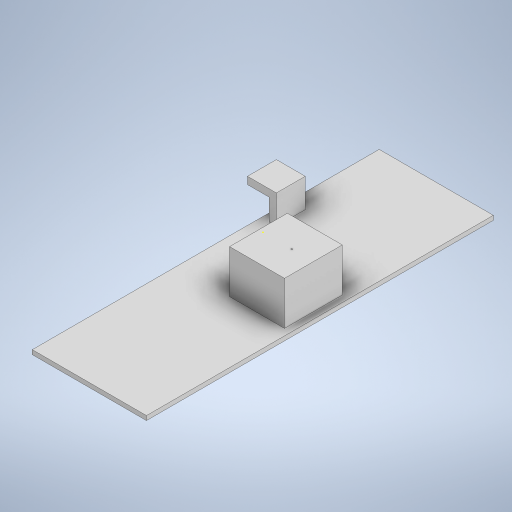
# Autodesk Inventor part: liquid port_v01
Saved by Autodesk Inventor 2023 (Build 270158000, 158)
## iProperties
Created: 2021-04-13
Part Number: liquid port_v01
Material: Generic
Document SubType Name: Modeling
Designer: KAMPFF-LAB-BEHAVIOR
Density: 1 g/cm^3
Appearance: Default
Author: KAMPFF-LAB-BEHAVIOR
Autodesk Inventor part; units mm, degrees
ref_plane "YZ Plane" through (0, 0, 0) normal (1, 0, 0) x (0, 1, 0)
ref_plane "XZ Plane" through (0, 0, 0) normal (0, 1, 0) x (-1, 0, 0)
ref_plane "XY Plane" through (0, 0, 0) normal (0, 0, 1) x (1, 0, 0)
sketch "Sketch44" plane through (0, 0, 0) normal (0, 1, 0) x (-1, 0, 0)
  line L0 (-39.5, 120) -> (39.5, 120)
  line L1 (39.5, 120) -> (39.5, -120)
  line L2 (39.5, -120) -> (-39.5, -120)
  line L3 (-39.5, -120) -> (-39.5, 120)
  line L4 (-39.5, 120) -> (39.5, -120) construction
  line L5 (39.5, 120) -> (-39.5, -120) construction
  point P0 (0, 0)
  dimension "d138" = 79
  dimension "d139" = 240
  constraints: 12 end point, 2 midpoint, 2 parallel, 1 horizontal, 1 perpendicular
  measures "d138" distance of L1.end L2.end
  measures "d139" distance of L0.end L1.end
extrude "Extrusion33" add sketch "Sketch44" along normal blind 3
sketch "Sketch45" plane through (0, 3, 0) normal (0, 1, 0) x (1, 0, 0)
  line L0 (35, -20) -> (-3, -20)
  line L1 (-3, -20) -> (-3, 20)
  line L2 (-3, 20) -> (35, 20)
  line L3 (35, 20) -> (35, -20)
  point P0 (0, 0)
  dimension "d142" = 38
  dimension "d143" = 40
  constraints: 8 end point, 2 parallel, 1 horizontal, 1 perpendicular
  measures "d142" distance of L1.end L2.end
  measures "d143" distance of L0.end L1.end
extrude "Extrusion34" add sketch "Sketch45" along normal blind 30
sketch "Sketch46" plane through (0, 33, 0) normal (0, 1, 0) x (1, 0, 0)
  point P0 (0, 0)
sketch "Sketch47" plane through (0, 0, 0) normal (0, -1, 0) x (1, 0, 0)
  circle A0 centre (16, 0) radius 18
  point P0 (0, 0)
  dimension "d146" = 36
  constraints: 1 centre point
  measures "d146" diameter of A0
extrude "Extrusion35" cut sketch "Sketch47" against normal blind 30 draft -15
sketch "Sketch48" plane through (0, 33, 0) normal (0, 1, 0) x (1, 0, 0)
  point P0 (0, 0)
sketch "Sketch49" plane through (0, 33, 0) normal (0, 1, 0) x (1, 0, 0)
  circle A0 centre (20, 0) radius 0.5
  point P0 (0, 0)
  dimension "d149" = 1
  constraints: 1 centre point
  measures "d149" diameter of A0
extrude "Extrusion36" cut sketch "Sketch49" against normal through all
sketch "Sketch58" plane through (35, 3, -20) normal (0, 0, -1) x (-1, 0, 0)
  line L0 (7, 20) -> (27, 20)
  line L1 (27, 20) -> (27, 5)
  line L2 (27, 5) -> (7, 5)
  line L3 (7, 5) -> (7, 20)
  point P0 (35, -3)
  dimension "d156" = 20
  dimension "d157" = 15
  constraints: 8 end point, 2 parallel, 1 horizontal, 1 perpendicular
  measures "d156" distance of L1.end L2.end
  measures "d157" distance of L0.end L1.end
extrude "Extrusion38" cut sketch "Sketch58" against normal blind 15
sketch "Sketch59" plane through (-3, 3, -20) normal (-1, 0, 0) x (0, 0, 1)
  line L0 (5, 25) -> (8, 25)
  line L1 (8, 25) -> (8, 5)
  line L2 (8, 5) -> (5, 5)
  line L3 (5, 5) -> (5, 25)
  point P0 (20, -3)
  dimension "d160" = 3
  dimension "d161" = 20
  constraints: 8 end point, 2 parallel, 1 horizontal, 1 perpendicular
  measures "d160" distance of L1.end L2.end
  measures "d161" distance of L0.end L1.end
extrude "Extrusion39" cut sketch "Sketch59" against normal blind 35
sketch "Sketch60" plane through (0, 3, 0) normal (0, 1, 0) x (1, 0, 0)
  line L0 (-33.965, 38.3247) -> (-28.965, 38.3247)
  line L1 (-28.965, 38.3247) -> (-28.965, 58.3247)
  line L2 (-28.965, 58.3247) -> (-33.965, 58.3247)
  line L3 (-33.965, 58.3247) -> (-33.965, 38.3247)
  point P0 (0, 0)
  dimension "d164" = 5
  dimension "d165" = 20
  constraints: 8 end point, 2 parallel, 1 horizontal, 1 perpendicular
  measures "d164" distance of L2.end L1.end
  measures "d165" distance of L1.end L0.end
extrude "Extrusion40" add sketch "Sketch60" along normal blind 20
sketch "Sketch61" plane through (0, 23, 0) normal (0, 1, 0) x (1, 0, 0)
  line L0 (-28.965, 38.3247) -> (-28.965, 58.3247) projected
  line L1 (-28.965, 38.3247) -> (-48.965, 38.3247)
  line L2 (-48.965, 38.3247) -> (-48.965, 58.3247)
  line L3 (-48.965, 58.3247) -> (-28.965, 58.3247)
  line L4 (-28.965, 58.3247) -> (-28.965, 38.3247)
  point P0 (0, 0)
  dimension "d168" = 20
  dimension "d169" = 20
  constraints: 8 end point, 2 parallel, 1 horizontal, 1 perpendicular
  measures "d168" distance of L2.end L3.end
  measures "d169" distance of L1.end L2.end
extrude "Extrusion41" add sketch "Sketch61" against normal blind 5
body "Solid9"
